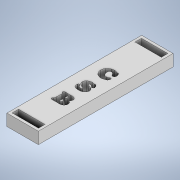
# Autodesk Inventor part: LegWithTextCSB
Saved by Autodesk Inventor 2021 (Build 250183000, 183)
## iProperties
Created: 2024-05-05
Part Number: LegWithTextCSB
Material: Generic
Document SubType Name: Modeling
Designer: brybr
Density: 1 g/cm^3
Appearance: Default
Author: brybr
Autodesk Inventor part; units mm, degrees
ref_plane "YZ Plane" through (0, 0, 0) normal (1, 0, 0) x (0, 1, 0)
ref_plane "XZ Plane" through (0, 0, 0) normal (0, 1, 0) x (-1, 0, 0)
ref_plane "XY Plane" through (0, 0, 0) normal (0, 0, 1) x (1, 0, 0)
sketch "Sketch1" plane through (0, 0, 0) normal (0, 0, 1) x (1, 0, 0)
  line L0 (-17.5, 6.5) -> (17.5, 6.5)
  line L1 (17.5, 6.5) -> (17.5, -6.5)
  line L2 (17.5, -6.5) -> (-17.5, -6.5)
  line L3 (-17.5, -6.5) -> (-17.5, 6.5)
  line L4 (-17.5, 6.5) -> (17.5, -6.5) construction
  line L5 (17.5, 6.5) -> (-17.5, -6.5) construction
  line L6 (-17.5, 6.5) -> (17.5, 6.5) construction
  point P0 (0, 0)
  dimension "d0" = 35
  dimension "d1" = 0
  dimension "d2" = 13
  constraints: 14 end point, 2 horizontal, 2 midpoint, 2 parallel, 1 collinear, 1 perpendicular
  measures "d0" distance of L0.start L0.end
  measures "d1" distance between parallel lines of L0 L6
  measures "d2" distance of L0.end L1.end
extrude "Extrusion1" add sketch "Sketch1" along normal blind 150
sketch "Sketch2" plane through (-17.5, 6.5, 0) normal (0, 1, 0) x (1, 0, 0)
  line L0 (2.8, -10.2) -> (32.2, -10.2)
  line L1 (32.2, -10.2) -> (32.2, -3)
  line L2 (32.2, -3) -> (2.8, -3)
  line L3 (2.8, -3) -> (2.8, -10.2)
  line L4 (2.8, -10.2) -> (32.2, -3) construction
  line L5 (32.2, -10.2) -> (2.8, -3) construction
  line L6 (2.8, -10.2) -> (32.2, -10.2) construction
  line L7 (2.8, -6.6) -> (0, -6.6)
  line L8 (0, 0) -> (0, -150) projected
  line L9 (35, 0) -> (35, -150) projected
  line L10 (35, -6.6) -> (32.2, -6.6)
  line L11 (35, 0) -> (0, 0) projected
  line L12 (2.8, -147) -> (32.2, -147)
  line L13 (32.2, -147) -> (32.2, -139.8)
  line L14 (32.2, -139.8) -> (2.8, -139.8)
  line L15 (2.8, -139.8) -> (2.8, -147)
  line L16 (2.8, -147) -> (32.2, -139.8) construction
  line L17 (32.2, -147) -> (2.8, -139.8) construction
  line L18 (2.8, -147) -> (32.2, -147) construction
  line L19 (2.8, -143.4) -> (0, -143.4)
  line L20 (35, -143.4) -> (32.2, -143.4)
  line L21 (35, -150) -> (0, -150) projected
  point P0 (17.5, 0)
  point P1 (17.5, -6.6)
  point P2 (17.5, -143.4)
  dimension "d6" = 29.4
  dimension "d7" = 0
  dimension "d8" = 7.2
  dimension "d9" = 3
  dimension "d12" = 29.4
  dimension "d13" = 0
  dimension "d14" = 7.2
  dimension "d15" = 3
  constraints: 36 end point, 8 midpoint, 6 horizontal, 6 point on line, 4 collinear, 4 parallel, 2 perpendicular
  measures "d6" distance of L0.start L0.end
  measures "d7" distance between parallel lines of L0 L6
  measures "d8" distance of L1.end L0.end
  measures "d9" distance between parallel lines of L11 L2
  measures "d12" distance of L12.start L12.end
  measures "d13" distance between parallel lines of L12 L18
  measures "d14" distance of L13.end L12.end
  measures "d15" distance between parallel lines of L21 L12
extrude "Extrusion2" cut sketch "Sketch2" against normal through all contours L3 L2 L1 L0 | L15 L14 L13 L12
sketch "Sketch3" plane through (-17.5, 6.5, 0) normal (0, 1, 0) x (1, 0, 0)
  line L0 (6.4393, -10.6292) -> (29.3125, -10.6292) construction
  line L1 (29.3125, -10.6292) -> (29.3125, -150.0931) construction
  line L2 (29.3125, -150.0931) -> (6.4393, -150.0931) construction
  line L3 (6.4393, -150.0931) -> (6.4393, -10.6292) construction
  spline S0 degree 2 poles (18.615, -48.7845) (20.1659, -48.7845) (21.6199, -49.4752) knots 0 0 0 1 1 1
  spline S1 degree 2 poles (21.6199, -49.4752) (22.2378, -49.7539) (22.4559, -49.7539) knots 0 0 0 1 1 1
  spline S2 degree 2 poles (22.4559, -49.7539) (22.6134, -49.7539) (23.0011, -49.669) knots 0 0 0 1 1 1
  spline S3 degree 2 poles (23.0011, -49.669) (23.1707, -49.6327) (23.3525, -49.6327) knots 0 0 0 1 1 1
  spline S4 degree 2 poles (23.3525, -49.6327) (23.9947, -49.6327) (24.4672, -50.2143) knots 0 0 0 1 1 1
  spline S5 degree 2 poles (24.4672, -50.2143) (25.5092, -51.4744) (25.5092, -53.3161) knots 0 0 0 1 1 1
  spline S6 degree 2 poles (25.5092, -53.3161) (25.5092, -54.6973) (24.552, -55.3395) knots 0 0 0 1 1 1
  spline S7 degree 2 poles (24.552, -55.3395) (24.031, -55.6787) (23.3888, -55.6787) knots 0 0 0 1 1 1
  spline S8 degree 2 poles (23.3888, -55.6787) (22.783, -55.6787) (22.0197, -55.1577) (21.6926, -54.5398) knots 0 0 0 1 2 2 2
  spline S9 degree 2 poles (21.6926, -54.5398) (21.2564, -53.728) (20.7233, -53.0495) (20.4082, -52.8193) knots 0 0 0 1 2 2 2
  spline S10 degree 2 poles (20.4082, -52.8193) (19.4026, -52.1165) (18.3727, -52.1165) knots 0 0 0 1 1 1
  spline S11 degree 2 poles (18.3727, -52.1165) (17.4155, -52.1165) (16.2766, -53.522) (16.2766, -54.7458) knots 0 0 0 1 2 2 2
  spline S12 degree 2 poles (16.2766, -54.7458) (16.2766, -56.4663) (17.1368, -57.896) knots 0 0 0 1 1 1
  spline S13 degree 2 poles (17.1368, -57.896) (18.3, -59.774) (20.4567, -59.774) knots 0 0 0 1 1 1
  spline S14 degree 2 poles (20.4567, -59.774) (21.2564, -59.774) (22.8194, -59.2409) (23.3525, -58.7563) knots 0 0 0 1 2 2 2
  spline S15 degree 2 poles (23.3525, -58.7563) (23.7039, -58.3928) (24.0431, -58.3928) knots 0 0 0 1 1 1
  spline S16 degree 2 poles (24.0431, -58.3928) (24.5157, -58.3928) (25.1336, -59.2167) (25.1336, -59.7498) knots 0 0 0 1 2 2 2
  spline S17 degree 2 poles (25.1336, -59.7498) (25.1336, -60.4041) (24.3703, -61.9913) (23.9098, -62.3548) knots 0 0 0 1 2 2 2
  spline S18 degree 2 poles (23.9098, -62.3548) (23.5706, -62.6456) (22.88, -62.791) knots 0 0 0 1 1 1
  spline S19 degree 2 poles (22.88, -62.791) (22.4559, -62.8637) (21.838, -63.1666) knots 0 0 0 1 1 1
  spline S20 degree 2 poles (21.838, -63.1666) (20.2507, -63.9178) (18.5544, -63.9178) knots 0 0 0 1 1 1
  spline S21 degree 2 poles (18.5544, -63.9178) (16.7612, -63.9178) (15.0043, -63.1303) knots 0 0 0 1 1 1
  spline S22 degree 2 poles (15.0043, -63.1303) (12.9446, -62.1973) (11.9632, -60.3799) knots 0 0 0 1 1 1
  spline S23 degree 2 poles (11.9632, -60.3799) (10.5819, -58.417) (10.5819, -56.3694) knots 0 0 0 1 1 1
  spline S24 degree 2 poles (10.5819, -56.3694) (10.5819, -53.9946) (12.048, -52.0438) knots 0 0 0 1 1 1
  spline S25 degree 2 poles (12.048, -52.0438) (13.3202, -50.3597) (15.38, -49.4631) knots 0 0 0 1 1 1
  spline S26 degree 2 poles (15.38, -49.4631) (16.9551, -48.7845) (18.615, -48.7845) knots 0 0 0 1 1 1
  spline S27 degree 2 poles (17.785, -72.8793) (18.8755, -72.8793) (20.6445, -73.4124) knots 0 0 0 1 1 1
  spline S28 degree 2 poles (20.6445, -73.4124) (20.8141, -73.473) (20.9111, -73.473) knots 0 0 0 1 1 1
  spline S29 degree 2 poles (20.9111, -73.473) (20.9716, -73.473) (21.4563, -73.3034) knots 0 0 0 1 1 1
  spline S30 degree 2 poles (21.4563, -73.3034) (21.6623, -73.2186) (21.8804, -73.2186) knots 0 0 0 1 1 1
  spline S31 degree 2 poles (21.8804, -73.2186) (22.6922, -73.2186) (24.34, -75.5691) (24.34, -76.6233) knots 0 0 0 1 2 2 2
  spline S32 degree 2 poles (24.34, -76.6233) (24.34, -77.2775) (23.5282, -78.2105) (22.9345, -78.2105) knots 0 0 0 1 2 2 2
  spline S33 degree 2 poles (22.9345, -78.2105) (22.4498, -78.2105) (21.8561, -77.8349) (20.9716, -77.011) knots 0 0 0 1 2 2 2
  spline S34 degree 2 poles (20.9716, -77.011) (19.7842, -75.9084) (18.6695, -75.9084) knots 0 0 0 1 1 1
  spline S35 degree 2 poles (18.6695, -75.9084) (18.1728, -75.9084) (17.6154, -76.3446) (17.6154, -76.696) knots 0 0 0 1 2 2 2
  spline S36 degree 2 poles (17.6154, -76.696) (17.6154, -77.4472) (19.1784, -77.8955) knots 0 0 0 1 1 1
  spline S37 degree 2 poles (19.1784, -77.8955) (21.2018, -78.5013) (21.8198, -78.7921) knots 0 0 0 1 1 1
  spline S38 degree 2 poles (21.8198, -78.7921) (24.5823, -80.137) (24.5823, -82.7662) knots 0 0 0 1 1 1
  spline S39 degree 2 poles (24.5823, -82.7662) (24.5823, -85.0805) (22.7043, -86.5344) knots 0 0 0 1 1 1
  spline S40 degree 2 poles (22.7043, -86.5344) (20.802, -88.0126) (17.7487, -88.0126) knots 0 0 0 1 1 1
  spline S41 degree 2 poles (17.7487, -88.0126) (16.3917, -88.0126) (13.3989, -87.3704) (12.6114, -86.8252) knots 0 0 0 1 2 2 2
  spline S42 degree 2 poles (12.6114, -86.8252) (12.151, -86.5465) (11.3149, -84.2323) (11.3149, -83.1176) knots 0 0 0 1 2 2 2
  spline S43 degree 2 poles (11.3149, -83.1176) (11.3149, -82.5481) (11.5209, -82.4027) knots 0 0 0 1 1 1
  spline S44 degree 2 poles (11.5209, -82.4027) (11.8844, -81.8212) (12.3933, -81.8212) knots 0 0 0 1 1 1
  spline S45 degree 2 poles (12.3933, -81.8212) (12.8779, -81.8212) (13.2657, -82.2452) knots 0 0 0 1 1 1
  spline S46 degree 2 poles (13.2657, -82.2452) (13.5443, -82.536) (14.3561, -83.7719) knots 0 0 0 1 1 1
  spline S47 degree 2 poles (14.3561, -83.7719) (14.7075, -84.3171) (16.2705, -85.032) (17.1186, -85.032) knots 0 0 0 1 2 2 2
  spline S48 degree 2 poles (17.1186, -85.032) (17.8214, -85.032) (18.6211, -84.5594) (18.6211, -84.2202) knots 0 0 0 1 2 2 2
  spline S49 degree 2 poles (18.6211, -84.2202) (18.6211, -83.9173) (17.991, -83.4084) (17.0338, -83.0934) knots 0 0 0 1 2 2 2
  spline S50 degree 2 poles (17.0338, -83.0934) (15.6889, -82.6935) (14.0896, -81.8817) (13.7624, -81.3365) knots 0 0 0 1 2 2 2
  spline S51 degree 2 poles (13.7624, -81.3365) (11.6905, -79.7614) (11.6905, -77.8228) knots 0 0 0 1 1 1
  spline S52 degree 2 poles (11.6905, -77.8228) (11.6905, -76.8535) (12.575, -75.0481) (13.3141, -74.4787) knots 0 0 0 1 2 2 2
  spline S53 degree 2 poles (13.3141, -74.4787) (15.1922, -72.8793) (17.785, -72.8793) knots 0 0 0 1 1 1
  line L4 (16.3493, -111.8166) -> (14.968, -111.8287)
  spline S54 degree 2 poles (14.968, -111.8287) (13.5262, -111.8529) (12.8719, -111.8893) knots 0 0 0 1 1 1
  spline S55 degree 2 poles (12.8719, -111.8893) (12.2539, -111.9377) (11.9753, -111.9377) knots 0 0 0 1 1 1
  spline S56 degree 2 poles (11.9753, -111.9377) (11.2604, -111.9377) (10.8363, -111.5864) knots 0 0 0 1 1 1
  spline S57 degree 2 poles (10.8363, -111.5864) (10.388, -111.1865) (10.388, -110.6413) knots 0 0 0 1 1 1
  spline S58 degree 2 poles (10.388, -110.6413) (10.388, -110.2778) (10.7152, -109.878) (11.2725, -109.4902) knots 0 0 0 1 2 2 2
  spline S59 degree 2 poles (11.2725, -109.4902) (11.5027, -109.3327) (11.7087, -108.5452) (11.842, -107.1033) knots 0 0 0 1 2 2 2
  spline S60 degree 2 poles (11.842, -107.1033) (12.0359, -104.8497) (12.0359, -101.5662) knots 0 0 0 1 1 1
  spline S61 degree 2 poles (12.0359, -101.5662) (12.0359, -100.403) (11.7572, -99.7124) (11.1514, -99.4458) knots 0 0 0 1 2 2 2
  spline S62 degree 2 poles (11.1514, -99.4458) (10.4365, -99.1429) (10.4365, -98.4402) knots 0 0 0 1 1 1
  spline S63 degree 2 poles (10.4365, -98.4402) (10.4365, -97.8828) (11.4058, -97.2043) (12.1207, -97.2043) knots 0 0 0 1 2 2 2
  spline S64 degree 2 poles (12.1207, -97.2043) (12.4236, -97.2043) (13.0415, -97.2406) knots 0 0 0 1 1 1
  spline S65 degree 2 poles (13.0415, -97.2406) (13.8654, -97.277) (14.9922, -97.277) knots 0 0 0 1 1 1
  spline S66 degree 2 poles (14.9922, -97.277) (15.8767, -97.277) (18.0334, -97.2164) knots 0 0 0 1 1 1
  spline S67 degree 2 poles (18.0334, -97.2164) (18.8695, -97.1922) (19.342, -97.1922) knots 0 0 0 1 1 1
  spline S68 degree 2 poles (19.342, -97.1922) (20.7354, -97.1922) (22.5165, -97.6647) (23.1707, -98.2221) knots 0 0 0 1 2 2 2
  spline S69 degree 2 poles (23.1707, -98.2221) (24.2612, -99.1429) (24.2612, -100.6696) knots 0 0 0 1 1 1
  spline S70 degree 2 poles (24.2612, -100.6696) (24.2612, -101.4329) (23.6191, -102.8869) (23.0617, -103.323) knots 0 0 0 1 2 2 2
  spline S71 degree 2 poles (23.0617, -103.323) (22.7951, -103.5411) (22.7951, -103.6744) knots 0 0 0 1 1 1
  spline S72 degree 2 poles (22.7951, -103.6744) (22.7951, -103.7956) (23.0859, -103.9167) knots 0 0 0 1 1 1
  spline S73 degree 2 poles (23.0859, -103.9167) (23.9947, -104.2802) (24.7095, -105.1284) knots 0 0 0 1 1 1
  spline S74 degree 2 poles (24.7095, -105.1284) (25.485, -106.0371) (25.485, -107.3578) knots 0 0 0 1 1 1
  spline S75 degree 2 poles (25.485, -107.3578) (25.485, -108.9329) (24.3339, -110.2293) knots 0 0 0 1 1 1
  spline S76 degree 2 poles (24.3339, -110.2293) (22.8315, -111.9377) (19.9236, -111.9377) knots 0 0 0 1 1 1
  spline S77 degree 2 poles (19.9236, -111.9377) (19.5237, -111.9377) (18.0213, -111.8772) knots 0 0 0 1 1 1
  spline S78 degree 2 poles (18.0213, -111.8772) (16.6522, -111.8287) (16.3493, -111.8166) knots 0 0 0 1 1 1
  line L5 (17.2943, -106.3279) -> (17.2943, -107.3093)
  spline S79 degree 2 poles (17.2943, -107.3093) (17.2943, -108.63) (17.6094, -109.357) (18.0698, -109.357) knots 0 0 0 1 2 2 2
  spline S80 degree 2 poles (18.0698, -109.357) (19.4268, -109.357) (19.4268, -107.7213) knots 0 0 0 1 1 1
  spline S81 degree 2 poles (19.4268, -107.7213) (19.4268, -105.6373) (17.8759, -105.6373) knots 0 0 0 1 1 1
  spline S82 degree 2 poles (17.8759, -105.6373) (17.5245, -105.6373) (17.2943, -105.8917) (17.2943, -106.3279) knots 0 0 0 1 2 2 2
  line L6 (17.2943, -100.3545) -> (17.2943, -102.4991)
  spline S83 degree 2 poles (17.2943, -102.4991) (17.2943, -102.9474) (17.4518, -103.214) (17.6457, -103.214) knots 0 0 0 1 2 2 2
  spline S84 degree 2 poles (17.6457, -103.214) (18.3121, -103.214) (18.93, -102.4022) (18.93, -101.4692) knots 0 0 0 1 2 2 2
  spline S85 degree 2 poles (18.93, -101.4692) (18.93, -100.5726) (18.2758, -99.6518) (17.7184, -99.6518) knots 0 0 0 1 2 2 2
  spline S86 degree 2 poles (17.7184, -99.6518) (17.464, -99.6518) (17.2943, -99.8941) (17.2943, -100.3545) knots 0 0 0 1 2 2 2
  point P0 (17.5, 0)
  constraints: 2 other
emboss "Emboss1" sketch "Sketch3" operation cut depth 20 direction (0, -1, 0)
sketch "Sketch4" plane through (-17.5, 6.5, 0) normal (0, 1, 0) x (1, 0, 0)
  line L0 (17.796, -111.9623) -> (18.61, -111.9623)
  line L1 (18.61, -111.9623) -> (18.61, -109.1669)
  line L2 (18.61, -109.1669) -> (17.796, -109.1669)
  line L3 (17.796, -109.1669) -> (17.796, -111.9623)
  line L4 (17.4202, -97.1682) -> (18.1771, -97.1682)
  line L5 (18.1771, -97.1682) -> (18.1771, -99.8895)
  line L6 (18.1771, -99.8895) -> (17.4202, -99.8895)
  line L7 (17.4202, -99.8895) -> (17.4202, -97.1682)
  point P0 (17.7184, -99.6518)
  point P1 (18.0334, -97.2164)
  constraints: 16 end point, 4 parallel, 2 horizontal, 2 perpendicular
extrude "Extrusion3" [suppressed]
body "Solid1"
